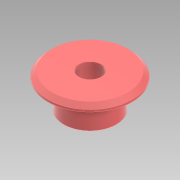
# Autodesk Inventor part: PocketPointBarPin
Saved by Autodesk Inventor 2021 (Build 250183000, 183)
## iProperties
Created: 2021-02-18
Part Number: PocketPointBarPin
Material: ABS プラスチック
Document SubType Name: Modeling
Designer: kumagai
Density: 1.06 g/cm^3
Appearance: 滑らか - 赤
Author: kumagai
Autodesk Inventor part; units mm, degrees
ref_plane "YZ Plane" through (0, 0, 0) normal (1, 0, 0) x (0, 1, 0)
ref_plane "XZ Plane" through (0, 0, 0) normal (0, 1, 0) x (-1, 0, 0)
ref_plane "XY Plane" through (0, 0, 0) normal (0, 0, 1) x (1, 0, 0)
sketch "スケッチ1" plane through (0, 0, 0) normal (0, 0, 1) x (1, 0, 0)
  line L0 (0, 0.64) -> (0, -3.84) projected
  line L1 (-0.8, 0) -> (4.8, 0) projected
  line L2 (1.05, 0) -> (1.05, -3.2)
  line L3 (1.05, -3.2) -> (2.5, -3.2)
  line L4 (2.5, -3.2) -> (2.5, -0.6)
  line L5 (2.5, -0.6) -> (4, -0.6)
  line L6 (4, -0.6) -> (4, 0)
  line L7 (4, 0) -> (1.05, 0)
  point P0 (0, 0)
  dimension "d0" = 1.05
  dimension "d1" = 2.5
  dimension "d2" = 3.2
  dimension "d3" = 2.6
  dimension "d4" = 4
  constraints: 12 end point, 5 perpendicular, 2 point on line, 1 vertical
  measures "d0" distance between parallel lines of L0 L2
  measures "d1" distance between parallel lines of L0 L4
  measures "d2" distance between parallel lines of L1 L3
  measures "d3" distance between parallel lines of L3 L5
  measures "d4" distance between parallel lines of L0 L6
revolve "回転1" add sketch "スケッチ1" angle 360 about axis through (0, 0, 0) along (0, -1, 0)
chamfer "面取り1" distance 0.4 angle 45 1 edges at (-4, 0, 0)
